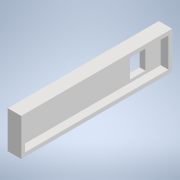
# Autodesk Inventor part: rearlightMount
Saved by Autodesk Inventor 2022.2 (Build 262287000, 287)
## iProperties
Created: 2022-04-24
Part Number: rearlightMount
Material: Generic
Document SubType Name: Modeling
Designer: foriw
Density: 1 g/cm^3
Appearance: Default
Author: foriw
Autodesk Inventor part; units mm, degrees
ref_plane "YZ Plane" through (0, 0, 0) normal (1, 0, 0) x (0, 1, 0)
ref_plane "XZ Plane" through (0, 0, 0) normal (0, 1, 0) x (-1, 0, 0)
ref_plane "XY Plane" through (0, 0, 0) normal (0, 0, 1) x (1, 0, 0)
sketch "Sketch1" plane through (0, 0, 0) normal (1, 0, 0) x (0, 1, 0)
  line L0 (-8, 37.75) -> (8, 37.75)
  line L1 (8, 37.75) -> (8, -37.75)
  line L2 (8, -37.75) -> (-8, -37.75)
  line L3 (-8, -37.75) -> (-8, 37.75)
  line L4 (-10, 39.75) -> (10, 39.75)
  line L5 (10, 39.75) -> (10, -39.75)
  line L6 (10, -39.75) -> (-10, -39.75)
  line L7 (-10, -39.75) -> (-10, 39.75)
  line L8 (-6.6198, 22.75) -> (6.3802, 22.75) construction
  line L9 (6.3802, 22.75) -> (6.3802, -19.25) construction
  line L10 (6.3802, -19.25) -> (-6.6198, -19.25) construction
  line L11 (-6.6198, -19.25) -> (-6.6198, 22.75) construction
  line L12 (-6.5, -21.75) -> (6.5, -21.75)
  line L13 (6.5, -21.75) -> (6.5, -29.75)
  line L14 (6.5, -29.75) -> (-6.5, -29.75)
  line L15 (-6.5, -29.75) -> (-6.5, -21.75)
  line L16 (8, 37.75) -> (-8, -37.75) construction
  line L17 (10, 39.75) -> (18, 39.75)
  line L18 (18, 39.75) -> (18, -39.75)
  line L19 (18, -39.75) -> (10, -39.75)
  line L20 (10, -39.75) -> (10, 39.75)
  line L21 (14, 29.75) -> (11, 29.75)
  line L22 (11, 29.75) -> (11, 23.75)
  line L23 (11, 23.75) -> (14, 23.75)
  line L24 (14, 23.75) -> (14, 29.75)
  line L25 (11, -20.25) -> (11, -26.25)
  line L26 (14, -26.25) -> (14, -20.25)
  line L27 (11, -26.25) -> (14, -26.25)
  line L28 (14, -20.25) -> (11, -20.25)
  point P0 (0, 0)
  point P1 (0, 0)
  point P2 (-3.5, 33.25)
  point P3 (3.5, -33.25)
  point P4 (0, 0)
  point P5 (14, 39.75)
  point P6 (12.5, 29.75)
  point P7 (10, -39.75)
  dimension "d0" = 16
  dimension "d1" = 75.5
  dimension "d2" = 4.5
  dimension "d3" = 4.5
  dimension "d4" = 2
  dimension "d5" = 4.5
  dimension "d6" = 4.5
  dimension "d7" = 13
  dimension "d8" = 42
  dimension "d9" = 15
  dimension "d10" = 13
  dimension "d11" = 8
  dimension "d12" = 1.5
  dimension "d13" = 16
  dimension "d18" = 8
  dimension "d19" = 3
  dimension "d20" = 6
  dimension "d23" = 50
  dimension "d28" = 10
  dimension "d40" = 4
  constraints: 58 end point, 12 parallel, 6 perpendicular, 5 horizontal, 3 midpoint, 1 coincident, 1 vertical, 11 other
  measures "d0" distance of L2.start L2.end
  measures "d1" distance of L1.start L2.start
  measures "d2" distance from line of L0 point (-3.5, 33.25)
  measures "d3" distance from line of L3 point (-3.5, 33.25)
  measures "d4" distance between parallel lines of L3 L7
  measures "d5" distance from line of point (3.5, -33.25) L2
  measures "d6" distance from line of point (3.5, -33.25) L1
  measures "d7" distance of L10.start L10.end
  measures "d8" distance of L9.start L10.start
  measures "d9" distance between parallel lines of L0 L8
  measures "d10" distance of L13.end L15.start
  measures "d11" distance of L13.start L13.end
  measures "d12" distance between parallel lines of L3 L15
  measures "d13" distance between parallel lines of L2 L12
  measures "d18" distance of L18.end L19.end
  measures "d19" distance of L23.end L22.end
  measures "d20" distance of L22.end L21.end
  measures "d23" distance of L21.end L25.start
  measures "d28" vertical distance of point (14, 39.75) point (12.5, 29.75)
  measures "d40" distance between parallel lines of L18 L24
extrude "Extrusion1" add sketch "Sketch1" against normal blind 3 contours L0 L1 L2 L3 | L4 L5 L6 L7
extrude "Extrusion2" add sketch "Sketch1" along normal blind 14 contours L4 L5 L6 L7
extrude "Extrusion3" add sketch "Sketch1" along normal blind 14 and the other way blind 3 contours L17 L18 L19 L5
hole "Hole1" at (0, 3.5, -33.25) at (0, -3.5, 33.25) direction (-1, 0, 0) diameter 3 end through all
fillet "Fillet1" radius 2 4 edges at (14, 14, 26.75) (14, 14, -23.25) (-3, 14, -23.25) (-3, 14, 26.75)
equation "\"d2\" = d3"
equation "\"d5\" = d3"
equation "\"d6\" = d3"
body "Solid1"
